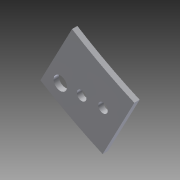
# Autodesk Inventor part: V5 Shooter Conveyor Spacer 1
Saved by Autodesk Inventor 2014 SP1 (Build 180222100, 222)
## iProperties
Created: 2012-03-01
Part Number: V5 Shooter Conveyor Spacer 1
Material: Aluminum-6061
Document SubType Name: Modeling
Designer: Moses
Density: 2.71 g/cm^3
Mass: 13.6538 g
Surface Area: 38.8978 cm^2
Volume: 5.03831 cm^3
Appearance: Aluminum - Flat
Author: Moses
Autodesk Inventor part; units mm, degrees
ref_plane "YZ Plane" through (0, 0, 0) normal (1, 0, 0) x (0, 1, 0)
ref_plane "XZ Plane" through (0, 0, 0) normal (0, 1, 0) x (-1, 0, 0)
ref_plane "XY Plane" through (0, 0, 0) normal (0, 0, 1) x (1, 0, 0)
sketch "Sketch1" plane through (0, 0, 0) normal (0, 0, 1) x (1, 0, 0)
  arc A0 (-24.5511, -4.3997) -> (12.4708, -23.8722) centre (142.4756, 268.2278) ccw
  line L0 (12.4708, -23.8722) -> (31.2882, 11.9043)
  arc A1 (-5.7336, 31.3768) -> (31.2882, 11.9043) centre (142.4756, 268.2278) ccw
  line L1 (-5.7336, 31.3768) -> (-24.5511, -4.3997)
  circle A2 centre (-12.7, 0) radius 4
  circle A3 centre (12.7, 0) radius 2.85
  circle A4 centre (0, 0) radius 2.85
  line L2 (-12.7, 0) -> (12.7, 0) construction
  dimension "d0" = 279.4
  dimension "d1" = 319.7243
  dimension "d2" = 25.4
  dimension "d3" = 40.4234
  dimension "d4" = 40.4234
  dimension "d8" = 31.3768
  dimension "d9" = 4.3997
  dimension "d10" = 18.5882
  dimension "d14" = 5.7
  dimension "d15" = 8
  constraints: 6 end point, 5 centre point, 4 point on circle, 2 coincident, 1 concentric, 1 equal radius, 1 horizontal, 1 midpoint, 1 parallel
  measures "d0" radius of A1
  measures "d1" radius of A0
  measures "d2" distance of L2.end L2.start
  measures "d3" distance of L1.start L1.end
  measures "d4" distance of L0.start L0.end
  measures "d8" distance from line of L2 L1.start
  measures "d9" distance from line of L1.end L2
  measures "d10" horizontal distance of L0.end L2.end
  measures "d14" diameter of A4
  measures "d15" diameter of A2
extrude "Extrusion1" add sketch "Sketch1" along normal blind 3.175
body "Solid1"
